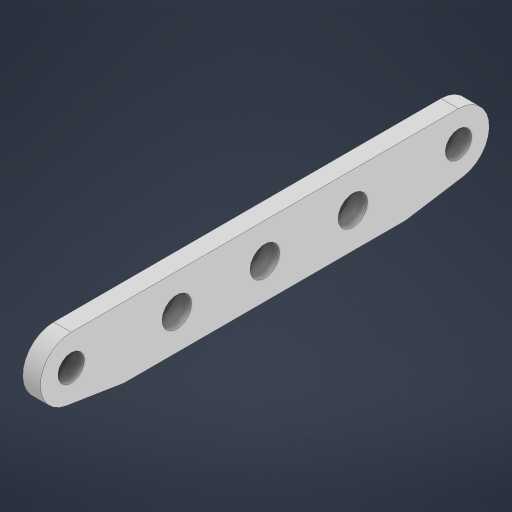
# Autodesk Inventor part: ElevatorCarriageBearingGusset
Saved by Autodesk Inventor 2023 (Build 270158000, 158)
## iProperties
Created: 2023-01-08
Part Number: ElevatorCarriageBearingGusset
Material: Generic
Document SubType Name: Modeling
Designer: Terrence
Density: 1 g/cm^3
Appearance: Default
Author: Terrence
Autodesk Inventor part; units mm, degrees
ref_plane "YZ Plane" through (0, 0, 0) normal (1, 0, 0) x (0, 1, 0)
ref_plane "XZ Plane" through (0, 0, 0) normal (0, 1, 0) x (-1, 0, 0)
ref_plane "XY Plane" through (0, 0, 0) normal (0, 0, 1) x (1, 0, 0)
sketch "Sketch1" plane through (0, 0, 0) normal (1, 0, 0) x (0, 1, 0)
  line L0 (0, 0) -> (12.7, 0)
  line L1 (12.7, 0) -> (12.7, -50.8)
  line L2 (12.7, -50.8) -> (0, -50.8)
  line L3 (0, -50.8) -> (0, 0)
  arc A0 (12.7, 9.525) -> (1.6567, 10.3991) centre (7.1437, 9.525) ccw
  line L4 (12.7, 0) -> (12.7, 9.525)
  line L5 (1.6567, 10.3991) -> (0, 0)
  line L6 (7.1437, 9.525) -> (7.1437, 0) construction
  circle A1 centre (7.1437, 9.525) radius 6.35 construction
  line L7 (12.7, -25.4) -> (0, -25.4) construction
  arc A2 (1.6567, -61.1991) -> (12.7, -60.325) centre (7.1438, -60.325) ccw
  line L8 (12.7, -50.8) -> (12.7, -60.325)
  line L9 (1.6567, -61.1991) -> (0, -50.8)
  circle A3 centre (7.1437, 9.525) radius 2.3813
  circle A4 centre (7.1438, -60.325) radius 2.3813
  dimension "d0" = 12.7
  dimension "d1" = 50.8
  dimension "d7" = 12.7
  dimension "d8" = 9.525
  dimension "d11" = 4.7625
  dimension "d25" = 3.175
  constraints: 20 end point, 5 centre point, 4 point on circle, 4 symmetric about line, 2 coincident, 2 midpoint, 2 parallel, 2 perpendicular, 2 tangent, 1 horizontal, 1 point on line, 1 vertical, 2 other
  measures "d0" distance of L1.end L2.end
  measures "d1" distance of L0.end L1.end
  measures "d7" diameter of A1
  measures "d8" distance of L6.start L6.end
  measures "d11" diameter of A3
  measures "d25" radial gap between concentric circles of A0 A3
extrude "Extrusion1" add sketch "Sketch1" along normal blind 3.175
sketch "Sketch2" plane through (3.175, 0, 0) normal (1, 0, 0) x (0, 0, -1)
  line L0 (60.325, 12.7) -> (-9.525, 12.7) projected
  line L1 (25.4, 12.7) -> (25.4, 0) construction
  line L2 (0, 0) -> (50.8, 0) projected
  line L3 (0, 12.7) -> (50.8, 12.7) construction
  line L4 (50.8, 12.7) -> (50.8, 38.1) construction
  line L5 (50.8, 38.1) -> (0, 38.1) construction
  line L6 (0, 38.1) -> (0, 12.7) construction
  line L7 (3.175, 34.925) -> (47.625, 34.925) construction
  line L8 (47.625, 34.925) -> (47.625, 15.875) construction
  line L9 (47.625, 15.875) -> (3.175, 15.875) construction
  line L10 (3.175, 15.875) -> (3.175, 34.925) construction
  circle A0 centre (9.525, 6.35) radius 2.667
  line L11 (25.4, 6.35) -> (44.9012, 6.35) construction
  circle A1 centre (25.4, 6.35) radius 2.667
  line L12 (9.525, 6.35) -> (32.9122, 6.35) construction
  circle A2 centre (41.275, 6.35) radius 2.667
  circle A3 centre (9.525, 6.35) radius 2.667
  circle A4 centre (25.4, 6.35) radius 2.667
  circle A5 centre (41.275, 6.35) radius 2.667
  dimension "d16" = 50.8
  dimension "d17" = 25.4
  dimension "d18" = 3.175
  dimension "d19" = 5.334
  dimension "d20" = 15.875
  dimension "d21" = 6.35
  dimension "d22" = 5.334
  constraints: 22 end point, 6 centre point, 4 midpoint, 4 parallel, 4 symmetric about line, 3 horizontal, 2 perpendicular, 2 point on line, 7 other
  measures "d16" distance of L4.end L5.end
  measures "d17" distance of L3.end L4.end
  measures "d18" distance between parallel lines of L5 L7
  measures "d19" diameter of A0
  measures "d20" distance from line of L1 L12.start
  measures "d21" distance from line of L0 L12.start
  measures "d22" diameter of A1
extrude "Extrusion2" cut sketch "Sketch2" against normal through all
fillet "Fillet1" radius 3.175 2 edges at (1.5875, 0, 0) (1.5875, 0, -50.8)
body "Solid1"
